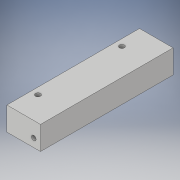
# Autodesk Inventor part: CupHolder
Saved by Autodesk Inventor 2019 (Build 230136000, 136)
## iProperties
Created: 2020-12-27
Part Number: CupHolder
Material: Типовые
Document SubType Name: Modeling
Designer: Professional
Density: 1 g/cm^3
Appearance: По умолчанию
Author: Professional
Autodesk Inventor part; units mm, degrees
ref_plane "YZ Plane" through (0, 0, 0) normal (1, 0, 0) x (0, 1, 0)
ref_plane "XZ Plane" through (0, 0, 0) normal (0, 1, 0) x (-1, 0, 0)
ref_plane "XY Plane" through (0, 0, 0) normal (0, 0, 1) x (1, 0, 0)
sketch "Эскиз1" plane through (0, 0, 0) normal (0, 0, 1) x (1, 0, 0)
  line L0 (-10, 0) -> (10, 0)
  line L1 (10, 0) -> (10, 14)
  line L2 (10, 14) -> (-10, 14)
  line L3 (-10, 14) -> (-10, 0)
  point P0 (0, 0)
  point P1 (0, 0)
  dimension "d0" = 20
  dimension "d1" = 14
  constraints: 8 end point, 2 parallel, 1 coincident, 1 horizontal, 1 midpoint, 1 perpendicular
  measures "d0" distance between parallel lines of L1 L3
  measures "d1" distance between parallel lines of L2 L0
extrude "Выдавливание1" add sketch "Эскиз1" along normal mid plane 79
sketch "Эскиз2" plane through (0, 0, 39.5) normal (0, 0, 1) x (1, 0, 0)
  circle A0 centre (6, 5) radius 1.4
  line L0 (-10, 0) -> (10, 0) projected
  line L1 (-10, 14) -> (-10, 0) projected
  point P0 (0, 0)
  point P1 (0, 0)
  dimension "d5" = 2.8
  dimension "d8" = 5
  dimension "d9" = 16
  constraints: 1 centre point, 1 midpoint
  measures "d5" diameter of A0
  measures "d8" distance from line of A0.centre L0
  measures "d9" distance from line of L1 A0.centre
extrude "Выдавливание2" cut sketch "Эскиз2" against normal blind 14
sketch "Эскиз3" plane through (-10, 0, -39.5) normal (-1, 0, 0) x (0, 0, 1)
  circle A0 centre (71.5, 5) radius 1.4
  circle A1 centre (7.5, 5) radius 1.4
  line L0 (39.5, 0) -> (79, 0) projected
  line L1 (0, 14) -> (79, 14) projected
  line L2 (39.5, 0) -> (39.5, 14)
  dimension "d10" = 64
  dimension "d11" = 5
  dimension "d12" = 2.8
  constraints: 2 centre point, 2 end point, 1 midpoint, 1 other
  measures "d10" distance of A0.centre A1.centre
  measures "d11" distance from line of L0 A1.centre
  measures "d12" diameter of A1
extrude "Выдавливание3" cut sketch "Эскиз3" against normal blind 16
mirror "Зеркальное отражение1" about plane through (0, 0, 0) normal (0, 0, 1) of "Выдавливание2"
sketch "Эскиз4" plane through (-10, 14, 39.5) normal (0, 1, 0) x (1, 0, 0)
  line L0 (0, 79) -> (0, 0) projected
  line L1 (0, 39.5) -> (20, 39.5)
  line L2 (20, 79) -> (20, 0) projected
  circle A0 centre (4, 64.5) radius 1.5
  circle A1 centre (4, 14.5) radius 1.5
  point P0 (10, 39.5)
  dimension "d15" = 50
  dimension "d16" = 3
  dimension "d17" = 4
  constraints: 2 centre point, 2 end point, 2 midpoint, 1 other
  measures "d15" distance of A0.centre A1.centre
  measures "d16" diameter of A0
  measures "d17" distance from line of L0 A0.centre
extrude "Выдавливание4" cut sketch "Эскиз4" against normal through all
sketch "Эскиз5" plane through (-10, 0, 39.5) normal (-1, 0, 0) x (0, 0, 1)
  line L0 (-67.3, 10) -> (-61.7, 10)
  line L1 (-61.7, 10) -> (-61.7, 7.4)
  line L2 (-61.7, 7.4) -> (-67.3, 7.4)
  line L3 (-67.3, 7.4) -> (-67.3, 10)
  line L4 (-39.5, 0) -> (-39.5, 14)
  line L5 (-79, 14) -> (0, 14) projected
  line L6 (-11.7, 10) -> (-17.3, 10)
  line L7 (-17.3, 10) -> (-17.3, 7.4)
  line L8 (-17.3, 7.4) -> (-11.7, 7.4)
  line L9 (-11.7, 7.4) -> (-11.7, 10)
  line L10 (-63, 0) -> (-66, 0) projected
  line L11 (-66, 14) -> (-63, 14) projected
  point P0 (-64.5, 7.4)
  point P1 (-64.5, 0)
  dimension "d20" = 5.6
  dimension "d21" = 4
  dimension "d22" = 2.6
  constraints: 18 end point, 4 symmetric about line, 3 midpoint, 2 parallel, 1 horizontal, 1 perpendicular, 1 vertical alignment
  measures "d20" distance of L0.start L0.end
  measures "d21" distance between parallel lines of L5 L0
  measures "d22" distance between parallel lines of L0 L2
extrude "Выдавливание5" cut sketch "Эскиз5" against normal blind 7
